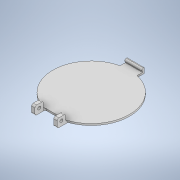
# Autodesk Inventor part: Tapacontenedor
Saved by Autodesk Inventor 2020.2 (Build 242310000, 310)
## iProperties
Created: 2020-10-22
Part Number: Tapacontenedor
Material: Generic
Document SubType Name: Modeling
Designer: JK
Density: 1 g/cm^3
Appearance: Default
Author: JK
Autodesk Inventor part; units mm, degrees
ref_plane "YZ Plane" through (0, 0, 0) normal (1, 0, 0) x (0, 1, 0)
ref_plane "XZ Plane" through (0, 0, 0) normal (0, 1, 0) x (-1, 0, 0)
ref_plane "XY Plane" through (0, 0, 0) normal (0, 0, 1) x (1, 0, 0)
sketch "Sketch1" plane through (0, 0, 0) normal (0, 1, 0) x (-1, 0, 0)
  circle A0 centre (0, 0) radius 45
  dimension "d0" = 90
  constraints: 1 centre point, 1 coincident
  measures "d0" diameter of A0
extrude "Extrusion1" add sketch "Sketch1" along normal blind 2
sketch "Sketch3" plane through (0, 0, 0) normal (1, 0, 0) x (0, 1, 0)
  line L0 (2, -45) -> (2, 45) projected
  line L1 (0, 15) -> (2, 15)
  line L2 (2, 15) -> (2, 55)
  line L3 (2, 55) -> (0, 55)
  line L4 (0, 55) -> (0, 15)
  line L5 (2, 55) -> (10, 55)
  line L6 (10, 55) -> (10, 45)
  line L7 (10, 45) -> (2, 45)
  line L8 (2, 45) -> (2, 55)
  point P0 (0, 0)
  point P1 (2, 15)
  point P2 (2, 45)
  dimension "d5" = 10
  dimension "d6" = 40
  dimension "d7" = 15
  dimension "d24" = 8
  constraints: 16 end point, 4 parallel, 2 horizontal, 2 perpendicular, 1 point on line
  measures "d5" distance of L5.end L6.end
  measures "d6" distance of L3.end L1.start
  measures "d7" distance from line of point (0, 0) L1
  measures "d24" distance of L2.end L5.end
extrude "Extrusion2" add sketch "Sketch3" along normal mid plane 30
sketch "Sketch4" plane through (-15, 10, 55) normal (0, 1, 0) x (1, 0, 0)
  line L0 (4, -4.8224) -> (26, -4.8224)
  line L1 (26, -4.8224) -> (26, 10)
  line L2 (26, 10) -> (4, 10)
  line L3 (4, 10) -> (4, -4.8224)
  line L4 (0, 0) -> (0, 10) projected
  line L5 (30, 10) -> (30, 0) projected
  line L6 (0, 10) -> (30, 10) projected
  point P0 (15, 55)
  dimension "d10" = 4
  dimension "d11" = 4
  constraints: 8 end point, 2 parallel, 1 collinear, 1 horizontal, 1 perpendicular
  measures "d10" distance between parallel lines of L4 L3
  measures "d11" distance between parallel lines of L5 L1
extrude "Extrusion3" cut sketch "Sketch4" against normal up to surface (8 mm away)
sketch "Sketch5" plane through (15, 0, 0) normal (1, 0, 0) x (0, 0, -1)
  circle A0 centre (-50, 5.5) radius 1.85
  line L0 (-45, 2) -> (-45, 10) projected
  line L1 (-45, 10) -> (-55, 10) projected
  point P0 (0, 0)
  dimension "d14" = 3.7
  dimension "d16" = 4.5
  dimension "d25" = 50
  constraints: 1 centre point
  measures "d14" diameter of A0
  measures "d16" distance from line of L1 A0.centre
  measures "d25" horizontal distance of point (0, 0) A0.centre
extrude "Extrusion4" cut sketch "Sketch5" against normal through all
sketch "Sketch6" plane through (0, 0, 0) normal (0, -1, 0) x (1, 0, 0)
  line L0 (-11, 43) -> (11, 43)
  line L1 (11, 43) -> (11, 71.9866)
  line L2 (11, 71.9866) -> (-11, 71.9866)
  line L3 (-11, 71.9866) -> (-11, 43)
  line L4 (-15, 42.4264) -> (-15, 55) projected
  line L5 (-15, 55) -> (15, 55) projected
  point P0 (0, 0)
  point P1 (11, 55)
  point P2 (-11, 55)
  dimension "d19" = 22
  dimension "d20" = 4
  dimension "d21" = 12
  constraints: 8 end point, 2 parallel, 1 horizontal, 1 perpendicular
  measures "d19" distance between parallel lines of L3 L1
  measures "d20" distance between parallel lines of L4 L3
  measures "d21" distance between parallel lines of L5 L0
extrude "Extrusion5" cut sketch "Sketch6" against normal through all contours L3 L5 L1 L0
fillet "Fillet1" radius 2 10 edges at (13, 2, 45) (13, 10, 45) (13, 10, 55) (13, 0, 55) (-11, 1, 43) (-13, 0, 55) (-13, 10, 55) (-13, 10, 45) (-13, 2, 45) (11, 1, 43)
sketch "Sketch7" plane through (0, 2, 0) normal (0, 1, 0) x (1, 0, 0)
  line L0 (10, 42) -> (-10, 42)
  line L1 (-10, 42) -> (-10, 50.2)
  line L2 (-10, 50.2) -> (10, 50.2)
  line L3 (10, 50.2) -> (10, 42)
  point P0 (0, 0)
  dimension "d27" = 10
  dimension "d28" = 20
  dimension "d31" = 8.2
  dimension "d32" = 42
  constraints: 8 end point, 2 parallel, 1 horizontal, 1 perpendicular
  measures "d27" distance from line of point (0, 0) L3
  measures "d28" distance of L1.end L2.end
  measures "d31" distance of L0.end L1.end
  measures "d32" distance from line of point (0, 0) L0
extrude "Extrusion6" add sketch "Sketch7" against normal blind 2
sketch "Sketch8" plane through (0, 0, 0) normal (0, -1, 0) x (1, 0, 0)
  line L0 (10, -43.8748) -> (10, -50.2) projected
  line L1 (10, -50.2) -> (-10, -50.2)
  line L2 (-10, -50.2) -> (-10, -52.2)
  line L3 (-10, -52.2) -> (10, -52.2)
  line L4 (10, -52.2) -> (10, -50.2)
  point P0 (0, 0)
  dimension "d33" = 2
  constraints: 8 end point, 2 parallel, 1 horizontal, 1 perpendicular
  measures "d33" distance between parallel lines of L3 L1
extrude "Extrusion7" add sketch "Sketch8" against normal blind 4
sketch "Sketch9" plane through (10, 0, -43.8748) normal (1, 0, 0) x (0, 0, -1)
  line L0 (6.3252, 4) -> (8.3252, 4) projected
  line L1 (8.3252, 4) -> (5.3252, 4)
  line L2 (5.3252, 4) -> (5.3252, 6)
  line L3 (5.3252, 6) -> (8.3252, 6)
  line L4 (8.3252, 6) -> (8.3252, 4)
  point P0 (-43.8748, 0)
  dimension "d36" = 2
  dimension "d37" = 3
  constraints: 8 end point, 2 parallel, 1 horizontal, 1 perpendicular
  measures "d36" distance between parallel lines of L3 L0
  measures "d37" distance of L2.end L3.end
extrude "Extrusion8" add sketch "Sketch9" against normal up to surface (20 mm away)
fillet "Fillet2" radius 2 1 edges at (0, 6, -49.2)
body "Solid1"
